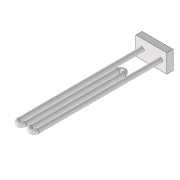
# Autodesk Inventor part: Heizwendel
Saved by Autodesk Inventor 2020 (Build 240168000, 168)
## iProperties
Created: 2020-04-08
Part Number: Heizwendel
Material: Generisch
Document SubType Name: Modeling
Designer: franz
Density: 1 g/cm^3
Appearance: Vorgabe
Author: franz
Autodesk Inventor part; units mm, degrees
ref_plane "YZ Plane" through (0, 0, 0) normal (1, 0, 0) x (0, 1, 0)
ref_plane "XZ Plane" through (0, 0, 0) normal (0, 1, 0) x (-1, 0, 0)
ref_plane "XY Plane" through (0, 0, 0) normal (0, 0, 1) x (1, 0, 0)
sketch "Skizze1" plane through (0, 0, 0) normal (0, 0, 1) x (1, 0, 0)
  line L0 (-25, -15) -> (25, -15)
  line L1 (25, -15) -> (25, 15)
  line L2 (25, 15) -> (-25, 15)
  line L3 (-25, 15) -> (-25, -15)
  line L4 (-25, -15) -> (25, 15) construction
  line L5 (25, -15) -> (-25, 15) construction
  point P0 (0, 0)
  dimension "d0" = 50
  dimension "d1" = 30
  constraints: 12 end point, 2 midpoint, 2 parallel, 1 horizontal, 1 perpendicular
  measures "d0" distance of L2.end L1.end
  measures "d1" distance of L1.end L0.end
extrude "Extrusion1" add sketch "Skizze1" along normal blind 10
sketch "Skizze2" plane through (0, 0, 10) normal (0, 0, 1) x (1, 0, 0)
  circle A0 centre (-15, 0) radius 3.5
  circle A1 centre (15, 0) radius 3.5
  line L0 (0, -21) -> (0, 21) projected
  point P0 (0, 0)
  dimension "d4" = 7
  dimension "d5" = 7
  dimension "d6" = 30
  constraints: 2 centre point, 1 symmetric about line
  measures "d4" diameter of A0
  measures "d5" diameter of A1
  measures "d6" distance of A1.centre A0.centre
sketch "Skizze3" plane through (0, 0, 0) normal (0, 1, 0) x (-1, 0, 0)
  line L0 (-25, 10) -> (25, 10) projected
  line L1 (-15, 10) -> (-15, 210)
  line L2 (15, 10) -> (15, 210)
  line L3 (5, 210) -> (5, 60)
  line L4 (-5, 60) -> (-5, 210)
  arc A0 (-5, 210) -> (-15, 210) centre (-10, 210) ccw
  arc A1 (15, 210) -> (5, 210) centre (10, 210) ccw
  arc A2 (-5, 60) -> (5, 60) centre (0, 60) ccw
  point P0 (0, 0)
  dimension "d7" = 30
  dimension "d8" = 15
  dimension "d9" = 200
  dimension "d10" = 200
  dimension "d11" = 150
  dimension "d12" = 10
  dimension "d13" = 10
  constraints: 8 end point, 6 point on circle, 6 tangent, 4 vertical, 3 centre point, 2 point on line
  measures "d7" distance between parallel lines of L2 L1
  measures "d8" distance from line of point (0, 0) L1
  measures "d9" distance of L1.start L1.end
  measures "d10" distance of L2.start L2.end
  measures "d11" distance of L4.start L4.end
  measures "d12" distance between parallel lines of L3 L2
  measures "d13" distance between parallel lines of L1 L4
sweep "Sweeping1" add profiles "Skizze2" path "Skizze3" separate body path curves L2 A1 L3 A2 L4 A0 L1 contours A0
equation "\"d10\" = d9"
